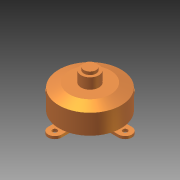
# Autodesk Inventor part: Lift_Motor
Saved by Autodesk Inventor 2011 SP1 (Build 150282100, 282)
## iProperties
Created: 2011-06-11
Part Number: Lift_Motor
Document SubType Name: Modeling
Designer: Andrew G. Meyer
Mass: 6.83252 g
Surface Area: 24.9795 cm^2
Volume: 6.83252 cm^3
Density: 1 g/cm^3
Author: Andrew G. Meyer
Autodesk Inventor part; units mm, degrees
ref_plane "YZ Plane" through (0, 0, 0) normal (1, 0, 0) x (0, 1, 0)
ref_plane "XZ Plane" through (0, 0, 0) normal (0, 1, 0) x (-1, 0, 0)
ref_plane "XY Plane" through (0, 0, 0) normal (0, 0, 1) x (1, 0, 0)
sketch "Sketch1" plane through (0, 0, 0) normal (0, 0, 1) x (1, 0, 0)
  line L0 (2.9264, -5.1404) -> (5.6442, -5.1404)
  line L1 (5.6442, -5.1404) -> (5.6442, -6.4866)
  line L2 (5.6442, -6.4866) -> (6.9015, -6.4866)
  line L3 (6.9015, -6.4866) -> (6.9015, -11.2364)
  line L4 (6.9015, -11.2364) -> (12.0958, -11.2364)
  line L5 (12.0958, -11.2364) -> (16.744, -13.1668)
  line L6 (16.744, -13.1668) -> (16.744, -22.006)
  line L7 (16.744, -22.006) -> (2.9264, -22.006)
  line L8 (2.9264, -22.006) -> (2.9264, -5.1404)
  point P0 (0, 0)
  dimension "d0" = 10.7696
  dimension "d1" = 8.8392
  dimension "d2" = 4.6482
  dimension "d3" = 13.8176
  dimension "d4" = 16.8656
  dimension "d5" = 1.3462
  dimension "d6" = 2.7178
  dimension "d7" = 3.9751
  constraints: 18 end point, 6 parallel, 1 horizontal, 1 perpendicular
  measures "d0" distance between parallel lines of L4 L7
  measures "d1" distance of L5.end L6.end
  measures "d2" horizontal distance of L5.end L4.end
  measures "d3" distance of L6.end L7.end
  measures "d4" distance of L7.end L0.start
  measures "d5" distance of L0.end L1.end
  measures "d6" distance of L0.start L0.end
  measures "d7" distance between parallel lines of L3 L8
revolve "Revolution1" add sketch "Sketch1" angle 360 about axis through (2.9264, -22.006, 0) along (0, 1, 0)
sketch "Sketch2" plane through (2.9264, -22.006, 0) normal (0, -1, 0) x (1, 0, 0)
  circle A0 centre (0, 0) radius 13.8176 projected
  line L0 (6.1468, 2.9718) -> (15.6464, 2.9718)
  line L1 (18.6182, 0) -> (18.6182, 0)
  line L2 (15.6464, -2.9718) -> (6.1468, -2.9718)
  line L3 (2.9718, 6.1468) -> (2.9718, 15.6464)
  line L4 (0, 18.6182) -> (0, 18.6182)
  line L5 (-2.9718, 15.6464) -> (-2.9718, 6.1468)
  line L6 (-6.1468, 2.9718) -> (-15.6464, 2.9718)
  line L7 (-18.6182, 0) -> (-18.6182, 0)
  line L8 (-15.6464, -2.9718) -> (-6.1468, -2.9718)
  line L9 (-2.9718, -6.1468) -> (-2.9718, -15.6464)
  line L10 (0, -18.6182) -> (0, -18.6182)
  line L11 (2.9718, -15.6464) -> (2.9718, -6.1468)
  arc A1 (-6.1468, 2.9718) -> (-2.9718, 6.1468) centre (-6.1468, 6.1468) ccw
  arc A2 (2.9718, 6.1468) -> (6.1468, 2.9718) centre (6.1468, 6.1468) ccw
  arc A3 (6.1468, -2.9718) -> (2.9718, -6.1468) centre (6.1468, -6.1468) ccw
  arc A4 (-2.9718, -6.1468) -> (-6.1468, -2.9718) centre (-6.1468, -6.1468) ccw
  arc A5 (18.6182, 0) -> (15.6464, 2.9718) centre (15.6464, 0) ccw
  arc A6 (15.6464, -2.9718) -> (18.6182, 0) centre (15.6464, 0) ccw
  arc A7 (2.9718, 15.6464) -> (0, 18.6182) centre (0, 15.6464) ccw
  arc A8 (0, 18.6182) -> (-2.9718, 15.6464) centre (0, 15.6464) ccw
  arc A9 (-15.6464, 2.9718) -> (-18.6182, 0) centre (-15.6464, 0) ccw
  arc A10 (-18.6182, 0) -> (-15.6464, -2.9718) centre (-15.6464, 0) ccw
  arc A11 (-2.9718, -15.6464) -> (0, -18.6182) centre (0, -15.6464) ccw
  arc A12 (0, -18.6182) -> (2.9718, -15.6464) centre (0, -15.6464) ccw
  circle A13 centre (0, 15.6464) radius 1.0668
  circle A14 centre (15.6464, 0) radius 1.0668
  circle A15 centre (-15.6464, 0) radius 1.0668
  circle A16 centre (0, -15.6464) radius 1.0668
  point P0 (-2.9264, 0)
  dimension "d9" = 3.175
  dimension "d10" = 5.9436
  dimension "d11" = 2.9718
  dimension "d12" = 5.9436
  dimension "d13" = 15.6464
  dimension "d14" = 15.6464
  dimension "d15" = 15.6464
  dimension "d16" = 2.1336
  constraints: 24 end point, 24 point on circle, 24 tangent, 16 centre point, 13 equal radius, 7 parallel, 6 perpendicular, 5 collinear, 4 coincident, 1 horizontal
  measures "d9" radius of A1
  measures "d10" distance between parallel lines of L2 L0
  measures "d11" radius of A5
  measures "d12" distance between parallel lines of L11 L9
  measures "d13" distance of A7.centre A0.centre
  measures "d14" distance of A5.centre A0.centre
  measures "d15" distance of A9.centre A0.centre
  measures "d16" diameter of A13
extrude "Extrusion1" add sketch "Sketch2" along normal blind 1.1684 contours A0 L2 A3 L11 L9 A4 L8 L6 A1 L5 L3 A2 L0 | A0 L0 A5 A6 L2 | A0 L5 A8 A7 L3 | L11 A12 A11 L9 A0 | A0 L8 A10 A9 L6
equation "\"d12\" = d10"
equation "\"d14\" = d13"
equation "\"d15\" = d13"
body "Solid1"
